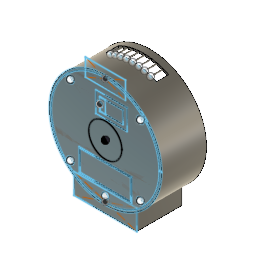
Whatscup design v6 (Autodesk Fusion 360 design; units mm, degrees)
Autodesk Fusion 360 part; units mm, degrees
sketch "Blueprint" plane through (0, 0, 0) normal (0, 1, 0) x (1, 0, 0)
  circle A0 centre (0, 0) radius 16.5
  line L0 (-25.1964, 19.7805) -> (25.2036, 19.7805)
  line L1 (25.2036, 19.7805) -> (25.2036, 40.3805)
  line L2 (25.2036, 40.3805) -> (-25.1964, 40.3805)
  line L3 (-25.1964, 40.3805) -> (-25.1964, 19.7805)
  line L4 (-5.4994, -34.7751) -> (17.6006, -34.7751)
  line L5 (17.6006, -34.7751) -> (17.6006, -22.2751)
  line L6 (17.6006, -22.2751) -> (-5.4994, -22.2751)
  line L7 (-5.4994, -22.2751) -> (-5.4994, -34.7751)
  line L8 (-5.4994, -34.7751) -> (0.0006, -34.7751)
  line L9 (0.0006, -34.7751) -> (0.0006, -22.2751)
  line L10 (0.0006, -22.2751) -> (-5.4994, -22.2751)
  line L11 (-5.4994, -22.2751) -> (-5.4994, -34.7751)
  line L12 (-31.4049, 42.8805) -> (31.4122, 42.8805)
  line L13 (31.4122, 42.8805) -> (31.4122, 63.421)
  line L14 (31.4122, 63.421) -> (-31.4049, 63.421)
  line L15 (-31.4049, 63.421) -> (-31.4049, 42.8805)
  line L16 (-31.4049, 42.8805) -> (31.4122, 63.421) construction
  line L17 (31.4122, 42.8805) -> (-31.4049, 63.421) construction
  circle A1 centre (-35, -35) radius 1.25
  circle A2 centre (35, -35) radius 1.25
  circle A3 centre (35, 35) radius 1.25
  circle A4 centre (-35, 35) radius 1.25
  line L18 (20.0006, -44.4682) -> (-19.9994, -44.4682)
  line L19 (-19.9994, -44.4682) -> (-19.9994, -61.8332)
  line L20 (-19.9994, -61.8332) -> (20.0006, -61.8332)
  line L21 (20.0006, -61.8332) -> (20.0006, -44.4682)
  line L22 (20.0006, -44.4682) -> (-19.9994, -61.8332) construction
  line L23 (-19.9994, -44.4682) -> (20.0006, -61.8332) construction
  circle A5 centre (0, 0) radius 53.9661
  line L24 (26.2036, 41.3805) -> (-26.1964, 41.3805)
  line L25 (-26.1964, 41.3805) -> (-26.1964, 18.7805)
  line L26 (-26.1964, 18.7805) -> (26.2036, 18.7805)
  line L27 (26.2036, 18.7805) -> (26.2036, 41.3805)
  circle A6 centre (0.0036, 48.0216) radius 2.8106
  line L28 (-9.4994, -38.7751) -> (21.6006, -38.7751)
  line L29 (21.6006, -38.7751) -> (21.6006, -18.2751)
  line L30 (21.6006, -18.2751) -> (-9.4994, -18.2751)
  line L31 (-9.4994, -18.2751) -> (-9.4994, -38.7751)
  line L32 (-7.4994, -26.7751) -> (-3.4994, -26.7751)
  line L33 (-3.4994, -26.7751) -> (-3.4994, -30.2751)
  line L34 (-3.4994, -30.2751) -> (-7.4994, -30.2751)
  line L35 (-7.4994, -30.2751) -> (-7.4994, -26.7751)
  line L36 (-7.4994, -26.7751) -> (-3.4994, -30.2751) construction
  line L37 (-3.4994, -26.7751) -> (-7.4994, -30.2751) construction
  circle A7 centre (35, -35) radius 3.25
  circle A8 centre (-35, -35) radius 3.25
  circle A9 centre (-35, 35) radius 3.25
  circle A10 centre (35, 35) radius 3.25
  point P0 (0.0036, 53.1507)
  point P1 (0.0006, -53.1507)
  point P2 (-5.4994, -28.5251)
  dimension "d1" = 33
  dimension "d2" = 50.4
  dimension "d3" = 20.6
  dimension "d4" = 23.1
  dimension "d5" = 12.5
  dimension "d6" = 5.5
  dimension "d7" = 12.5
  dimension "d9" = 2.5
  dimension "d10" = 2.5
  dimension "d11" = 2.5
  dimension "d12" = 2.5
  dimension "d13" = 40
  dimension "d36" = 1
  dimension "d43" = 5.6212
  dimension "d44" = 4
  dimension "d47" = 4
  dimension "d48" = 3.5
  dimension "d68" = 2
  dimension "d69" = 2
  dimension "d70" = 2
  dimension "d71" = 2
  constraint coincident A0.centre A5.centre
  constraint horizontal L0
  constraint vertical L1
  constraint horizontal L2
  constraint vertical L3
  constraint horizontal L4
  constraint vertical L5
  constraint horizontal L6
  constraint vertical L7
  constraint horizontal L8
  constraint vertical L9
  constraint horizontal L10
  constraint vertical L11
  constraint horizontal L12
  constraint perpendicular L12 L13
  constraint parallel L12 L14
  constraint parallel L13 L15
  constraint coincident L16 P0
  constraint coincident L17 P0
  constraint horizontal L18
  constraint perpendicular L18 L19
  constraint parallel L18 L20
  constraint parallel L19 L21
  constraint coincident L22 P1
  constraint coincident L23 P1
  constraint concentric A0 A5
  constraint horizontal L32
  constraint perpendicular L32 L33
  constraint parallel L32 L34
  constraint parallel L33 L35
  constraint coincident L36 P2
  constraint coincident L37 P2
  constraint midpoint L7 P2
  measures "d1" diameter of A0
  measures "d2" distance of L0.start L0.end
  measures "d3" distance of L0.start L2.end
  measures "d4" distance of L4.start L4.end
  measures "d5" distance of L4.start L6.end
  measures "d6" distance of L4.start L8.end
  measures "d7" distance of L4.start L6.end
  measures "d9" diameter of A1
  measures "d10" diameter of A2
  measures "d11" diameter of A3
  measures "d12" diameter of A4
  measures "d13" distance of L19.end L20.end
  measures "d43" diameter of A6
  measures "d47" distance of L33.end L34.end
  measures "d48" distance of L32.end L33.end
sketch "Shell" plane through (0, 0, 0) normal (0, 1, 0) x (1, 0, 0)
  circle A0 centre (0, 0) radius 54.0833
  circle A1 centre (0, 0) radius 56.0833
  dimension "d29" = 2
  constraint coincident A0.centre A1.centre
extrude "Extrude6" add sketch "Shell" along normal blind 30 contours A1 picked at (-42.3653, 35.5084) makes body 1
extrude "Extrude7" add sketch "Shell" along normal blind 2 contours A0 picked at (6.4276, -1.8327) bodies 1
extrude "Extrude8" add sketch "Blueprint" along normal blind 30 separate body contours L13 L14 L15 A5 picked at (-1.2367, 60.2266) makes body 2
extrude "Extrude9" add sketch "Blueprint" along normal blind 15 separate body contours L24 L25 L26 L27 picked at (-8.3964, 41.0471) makes body 3
sketch "Huzzah port" plane through (26.2036, 0, 0) normal (1, 0, 0) x (0, 1, 0)
  line L0 (0, -18.7805) -> (0, -41.3805)
  line L1 (0, -41.3805) -> (15, -41.3805)
  line L2 (15, -41.3805) -> (15, -18.7805)
  line L3 (15, -18.7805) -> (0, -18.7805)
  arc A0 (2, -37.6755) -> (2, -24.3245) centre (2, -31) ccw
  line L4 (2, -24.3245) -> (2, -37.6755)
  constraint vertical L4
extrude "Extrude10" cut sketch "Huzzah port" against normal blind 1 contours A0 L4 picked at (4.479, -33.5988) bodies 3
extrude "Extrude11" cut sketch "Blueprint" along normal blind 2 contours A6 picked at (-1.5811, 47.4331) bodies 1
extrude "Extrude12" add sketch "Blueprint" along normal blind 19 separate body contours L7 L11 L32 L34 L35 | L28 L29 L30 L31 picked at (-6.166, -29.1084) picked at (4.034, -19.6084) makes body 4
sketch "Sketch4" plane through (0, 19, 0) normal (0, 1, 0) x (-1, 0, 0)
  line L0 (5.4994, 34.7751) -> (5.4994, 22.2751)
  line L1 (5.4994, 22.2751) -> (-17.6006, 22.2751)
  line L2 (-17.6006, 22.2751) -> (-17.6006, 34.7751)
  line L3 (-17.6006, 34.7751) -> (5.4994, 34.7751)
  line L4 (9.4994, 18.2751) -> (9.4994, 38.7751)
  line L5 (9.4994, 38.7751) -> (-21.6006, 38.7751)
  line L6 (-21.6006, 38.7751) -> (-21.6006, 18.2751)
  line L7 (-21.6006, 18.2751) -> (9.4994, 18.2751)
  line L8 (3.4994, 26.7751) -> (7.4994, 26.7751)
  line L9 (7.4994, 26.7751) -> (7.4994, 30.2751)
  line L10 (7.4994, 30.2751) -> (3.4994, 30.2751)
  line L11 (3.4994, 30.2751) -> (3.4994, 26.7751)
  line L12 (3.4994, 26.7751) -> (7.4994, 30.2751) construction
  line L13 (7.4994, 26.7751) -> (3.4994, 30.2751) construction
  point P0 (5.4994, 28.5251)
  dimension "d49" = 4
  dimension "d50" = 3.5
  constraint horizontal L8
  constraint perpendicular L8 L9
  constraint parallel L8 L10
  constraint parallel L9 L11
  constraint coincident L12 P0
  constraint coincident L13 P0
  constraint midpoint L0 P0
  measures "d49" distance of L9.end L10.end
  measures "d50" distance of L8.end L9.end
extrude "Extrude13" cut sketch "Sketch4" against normal blind 17 contours L0 L8 L9 L10 picked at (6.166, 29.1084) bodies 4
sketch "Sketch5" plane through (-9.4994, 0, 0) normal (-1, 0, 0) x (0, -1, 0)
  line L0 (0, 18.2751) -> (0, 38.7751)
  line L1 (0, 38.7751) -> (-19, 38.7751)
  line L2 (-19, 38.7751) -> (-19, 18.2751)
  line L3 (-19, 18.2751) -> (0, 18.2751)
  line L4 (-2, 25) -> (-15.1103, 25)
  line L5 (-15.1103, 25) -> (-15.1103, 32.0501)
  line L6 (-15.1103, 32.0501) -> (-2, 32.0501)
  line L7 (-2, 32.0501) -> (-2, 25)
  line L8 (-2, 25) -> (-15.1103, 32.0501) construction
  line L9 (-15.1103, 25) -> (-2, 32.0501) construction
  point P0 (-8.5551, 28.5251)
  constraint horizontal L4
  constraint perpendicular L4 L5
  constraint parallel L4 L6
  constraint parallel L5 L7
  constraint coincident L8 P0
  constraint coincident L9 P0
extrude "Extrude14" cut sketch "Sketch5" against normal blind 5 contours L4 L5 L6 L7 picked at (-6.3701, 27.35) bodies 4
extrude "Extrude15" add sketch "Shell" along normal blind 45 separate body contours A1 picked at (-42.3653, 35.5084) makes body 5
extrude "Extrude16" add sketch "Blueprint" along normal blind 45 separate body contours L13 L14 L15 A5 picked at (-1.2367, 60.2266) makes body 6
extrude "Extrude17" add sketch "Shell" along normal blind 2 separate body contours A0 picked at (6.4276, -1.8327) makes body 7
ref_plane "WorkPlane2" through (6.0506, 26, 28.5251) normal (0, 1, 0) x (0, 0, 1)
box "BoxPrimitive1" cut length 17 width 50 height 12 placed x (0, 0, -1) y (-1, 0, 0) z (0, 1, 0) at (25.0506, 26, 61.5251) bodies 5
extrude "Extrude18" add sketch "Blueprint" along normal blind 45 separate body contours A7 picked at (37.5712, -35.1615) makes body 8
extrude "Extrude19" add sketch "Blueprint" along normal blind 45 separate body contours A8 picked at (-32.4334, -35.2236) makes body 9
extrude "Extrude20" add sketch "Blueprint" along normal blind 45 separate body contours A9 picked at (-32.4288, 34.8385) makes body 10
extrude "Extrude21" add sketch "Blueprint" along normal blind 45 separate body contours A10 picked at (37.5712, 34.8385) makes body 11
sketch "Sketch7" plane through (0, 26, 0) normal (0, 1, 0) x (-1, 0, 0)
  arc A0 (24.9494, 47.9847) -> (-25.0506, 47.9319) centre (0, 0) ccw
  line L0 (24.9494, 47.9847) -> (24.9494, 50.2281)
  arc A1 (24.9494, 50.2281) -> (-25.0506, 50.1777) centre (0, 0) ccw
  line L1 (-25.0506, 50.1777) -> (-25.0506, 47.9319)
  circle A2 centre (-19.009, 51.4644) radius 0.8
  circle A3 centre (-12.9813, 53.3233) radius 0.8
  circle A4 centre (-7.2698, 54.3997) radius 0.8
  circle A5 centre (-1.0673, 54.8831) radius 0.8
  circle A6 centre (4.9659, 54.6581) radius 0.8
  circle A7 centre (10.837, 53.8027) radius 0.8
  circle A8 centre (16.1951, 52.4394) radius 0.8
  circle A9 centre (21.1597, 50.6403) radius 0.8
  dimension "d80" = 1.6
  dimension "d81" = 1.6
  dimension "d82" = 1.6
  dimension "d83" = 1.6
  dimension "d84" = 1.6
  dimension "d85" = 1.6
  dimension "d86" = 1.6
  dimension "d87" = 1.6
  measures "d80" diameter of A2
  measures "d81" diameter of A3
  measures "d82" diameter of A4
  measures "d83" diameter of A5
  measures "d84" diameter of A6
  measures "d85" diameter of A7
  measures "d86" diameter of A8
  measures "d87" diameter of A9
extrude "Extrude22" add sketch "Sketch7" along normal blind 12 contours A0 A2 picked at (-18.9169, 51.2286) bodies 5
extrude "Extrude23" add sketch "Sketch7" along normal blind 12 contours A0 A3 picked at (-13.0695, 53.5754) bodies 5
extrude "Extrude24" add sketch "Sketch7" along normal blind 12 contours A4 picked at (-6.8326, 54.6342) bodies 5
extrude "Extrude25" add sketch "Sketch7" along normal blind 12 contours A5 picked at (-0.7531, 55.0645) bodies 5
extrude "Extrude26" add sketch "Sketch7" along normal blind 12 contours A6 picked at (5.1915, 54.5205) bodies 5
extrude "Extrude27" add sketch "Sketch7" along normal blind 12 contours A7 picked at (11.2034, 54.0161) bodies 5
extrude "Extrude28" add sketch "Sketch7" along normal blind 12 contours A8 picked at (15.9369, 52.7609) bodies 5
extrude "Extrude29" add sketch "Sketch7" along normal blind 12 contours A9 picked at (21.4186, 50.8328) bodies 5
hidden bodies 1 2
